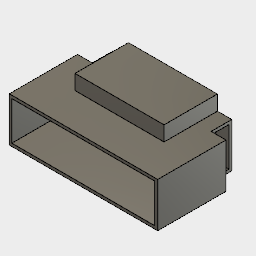
keyWithMesh (Autodesk Fusion 360 design; units mm, degrees)
Autodesk Fusion 360 part; units mm, degrees
sketch "スケッチ1" plane through (0, 0, 0) normal (0, 1, 0) x (1, 0, 0)
  line L0 (-25, 10) -> (25, 10)
  line L1 (25, 10) -> (25, -20)
  line L2 (25, -20) -> (-25, -20)
  line L3 (-25, -20) -> (-25, 10)
  dimension "d1" = 50
  measures "d1" distance of L0.start L0.end
extrude "押し出し1" add sketch "スケッチ1" along normal blind 15
sketch "スケッチ2" plane through (0, 0, 20) normal (0, 0, 1) x (1, 0, 0)
  line L0 (-25, 0) -> (25, 0)
  line L1 (25, 0) -> (25, 15)
  line L2 (25, 15) -> (-25, 15)
  line L3 (-25, 15) -> (-25, 0)
  line L4 (-24.1188, 14.0157) -> (23.8812, 14.0157)
  line L5 (23.8812, 14.0157) -> (23.8812, 1.0157)
  line L6 (23.8812, 1.0157) -> (-24.1188, 1.0157)
  line L7 (-24.1188, 1.0157) -> (-24.1188, 14.0157)
  dimension "d4" = 48
  dimension "d5" = 13
  measures "d4" distance of L4.start L4.end
  measures "d5" distance of L4.start L6.end
extrude "押し出し2" cut sketch "スケッチ2" against normal blind 29 contours L4 L5 L6 L7
sketch "スケッチ3" plane through (0, 15, 0) normal (0, 1, 0) x (-1, 0, 0)
  line L0 (25, 20) -> (-25, 20)
  line L1 (-25, 20) -> (-25, -10)
  line L2 (-25, -10) -> (25, -10)
  line L3 (25, -10) -> (25, 20)
  line L4 (25, -10) -> (20, -10)
  line L5 (20, -10) -> (20, -3)
  line L6 (20, -3) -> (25, -3)
  line L7 (25, -3) -> (25, -10)
  dimension "d8" = 5
  dimension "d9" = 7
  measures "d8" distance of L2.end L4.end
  measures "d9" distance of L2.end L6.end
extrude "押し出し3" cut sketch "スケッチ3" against normal blind 25 contours L2 L3 L4 L5 L6 L7
sketch "スケッチ4" plane through (0, 15, 0) normal (0, 1, 0) x (-1, 0, 0)
  line L0 (20, -10) -> (20, -3)
  line L1 (20, -3) -> (25, -3)
  line L2 (25, -3) -> (25, 20)
  line L3 (25, 20) -> (-25, 20)
  line L4 (-25, 20) -> (-25, -10)
  line L5 (-25, -10) -> (20, -10)
  line L6 (-25, -10) -> (-20, -10)
  line L7 (-20, -10) -> (-20, -3)
  line L8 (-20, -3) -> (-25, -3)
  line L9 (-25, -3) -> (-25, -10)
  dimension "d12" = 7
  dimension "d13" = 5
  measures "d12" distance of L4.end L8.end
  measures "d13" distance of L4.end L6.end
extrude "押し出し4" cut sketch "スケッチ4" against normal blind 65 contours L4 L5 L6 L7 L8 L9
sketch "スケッチ5" plane through (0, 15, 0) normal (0, 1, 0) x (-1, 0, 0)
  line L0 (-25, -3) -> (-20, -3)
  line L1 (-20, -3) -> (-20, -10)
  line L2 (-20, -10) -> (20, -10)
  line L3 (20, -10) -> (20, -3)
  line L4 (20, -3) -> (25, -3)
  line L5 (25, -3) -> (25, 20)
  line L6 (25, 20) -> (-25, 20)
  line L7 (-25, 20) -> (-25, -3)
  line L8 (14.8509, -10) -> (-15.1491, -10)
  line L9 (-15.1491, -10) -> (-15.1491, 8)
  line L10 (-15.1491, 8) -> (14.8509, 8)
  line L11 (14.8509, 8) -> (14.8509, -10)
  dimension "d16" = 30
  dimension "d17" = 18
  measures "d16" distance of L8.start L8.end
  measures "d17" distance of L8.start L10.end
extrude "押し出し5" add sketch "スケッチ5" along normal blind 5 contours L2 L8 L9 L10 L11
